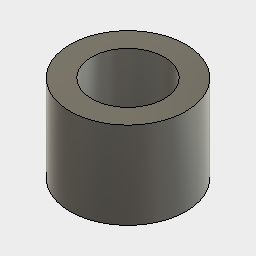
Shaft alignment guide (Autodesk Fusion 360 design; units mm, degrees)
Autodesk Fusion 360 part; units mm, degrees
sketch "Sketch1" plane through (0, 0, 0) normal (0, 1, 0) x (1, 0, 0)
  circle A0 centre (0, 0) radius 3 construction
  circle A1 centre (0, 0) radius 2.5 construction
  circle A2 centre (0, 0) radius 4 construction
  dimension "d1" = 6
  dimension "d2" = 5
  dimension "d3" = 8
  constraint coincident A0.centre A1.centre
  measures "d1" diameter of A0
  measures "d2" diameter of A1
  measures "d3" diameter of A2
sketch "Sketch2" plane through (0, 0, 0) normal (0, 1, 0) x (1, 0, 0)
  circle A0 centre (0, 0) radius 3
  circle A1 centre (0, 0) radius 3
  circle A2 centre (0, 0) radius 4
  circle A3 centre (0, 0) radius 4
  circle A4 centre (0, 0) radius 4
  circle A5 centre (0, 0) radius 3
  constraint coincident A0.centre A1.centre
  constraint equal A2 A4
  constraint equal A0 A5
extrude "Extrude1" add sketch "Sketch2" along normal blind 2
sketch "Sketch3" plane through (0, 2, 0) normal (0, 1, 0) x (-1, 0, 0)
  circle A0 centre (0, 0) radius 3
  circle A1 centre (0, 0) radius 4
  circle A2 centre (0, 0) radius 2.5
  circle A3 centre (0, 0) radius 4
  circle A4 centre (0, 0) radius 4
  circle A5 centre (0, 0) radius 2.5
  constraint coincident A0.centre A1.centre
  constraint equal A3 A4
  constraint equal A2 A5
extrude "Extrude2" add sketch "Sketch3" along normal blind 4 contours A0 | A1 A3 A4
